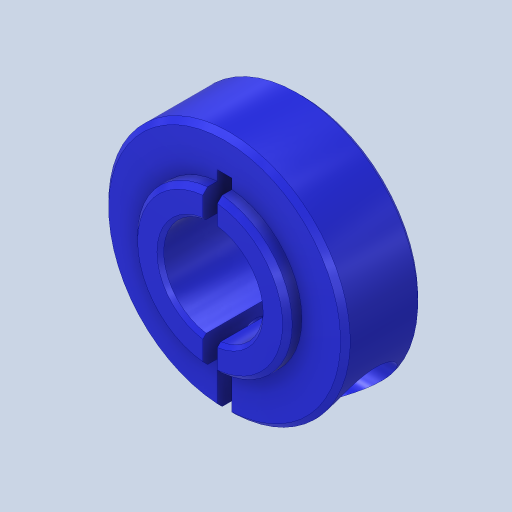
# Autodesk Inventor part: SCBNJ10-16b
Saved by Autodesk Inventor 2024 (Build 280153000, 153)
## iProperties
Category: PARTsolutions
Company: MISUMI
Created: 2024-03-13
Part Number: SCBNJ10-16b
Material: ABS プラスチック
Catalog Web Link: www.cadenas.de
Description: SCBNJ, PSCBNJ, SSCBNJ, SCSNAJ, SCSNAWJ, SCLSJ, PSCLSJ, SSCLSJ-b-Set Collars - For Bearing Fixing - Slit Compact Type
Vendor: MISUMI
Document SubType Name: Modeling
Designer: psAdmin
Manufacturer: MISUMI
Mass: 3.07278 g
Surface Area: 20.4444 cm^2
Volume: 3.07278 cm^3
Density: 1.06 g/cm^3
Appearance: 青 - 壁塗料 - 光沢
PSOL_IDENT_0: {$CADENAS_DATA/23d-libs/misumi/metric/03_set_collars/scbnj_b.prj},235 {VTYP=3D},{NB=SCBNJ10-16b},{LI
PSOL_IDENT_1: NA=SCBNJ10-16b},{NN=SCBNJ, PSCBNJ, SSCBNJ, SCSNAJ, SCSNAWJ, SCLSJ, PSCLSJ, SSCLSJ-b},{DATE=31.05.202
PSOL_IDENT_2: 3 07:34:13},{GEOMDATE=14.04.2023 07:53:48},{VERSION=},{LINEID=60},{WBVAR=TS,MAT,ST,DSS},{WBNUMERIC=D
PSOL_IDENT_3: SS}  {NB=SCBNJ10-16b},{LINA=SCBNJ10-16b},{KT=DUMMY},{PN=SCBNJ10-16},{TYPE=SCBNJ},{D=10},{TS=SN},{TS1='
PSOL_IDENT_4: SN','Short Nose','LN','Long Nose'},{MAT=1045},{MATA='1045','1045 Carbon Steel','304','304 Stainless
PSOL_IDENT_5: Steel','2017','2017 Aluminum Alloy'},{ST=Black Oxide},{ST0='Black Oxide','Black Oxide','Electroless
PSOL_IDENT_6: Nickel Plating','Electroless Nickel Plating'},{DSS=16},{DS1=13,14,16},{AC=Set Screws 2 Pcs.},{AB=620
PSOL_IDENT_7: 0ZZ(30)-6300ZZ(35)},{B=9.5},{B1=12.0},{D1=25},{M=M3},{THMD=3},{BB=8.0},{C=0.5},{L=10},{DD=3.5},{R=3.
PSOL_IDENT_8: 00},{W=1.5},{X=8.0},{Y=4.0},{Z=9.000},{COLOR=0.00,0.00,0.00,0.00}
NB: SCBNJ10-16b
NN: SCBNJ, PSCBNJ, SSCBNJ, SCSNAJ, SCSNAWJ, SCLSJ, PSCLSJ, SSCLSJ-b
NT: Set Collars - For Bearing Fixing - Slit Compact Type
NBSYN: $PN.b
LINA: SCBNJ10-16b
CATALOG: Misumi
PN: SCBNJ10-16
D: 10
TS: Short Nose
MAT: 1045 Carbon Steel
ST: Black Oxide
DSS: 16
AC: Set Screws 2 Pcs.
AB: 6200ZZ(30)-6300ZZ(35)
B: 9.5
B1: 12
D1: 25
M: M3
BB: 8
C: 0.5
L: 10
DD: 3.5
R: 3
W: 1.5
X: 8
Y: 4
Z: 9
SUPPLIER: MISUMI
ARTICLENO: SCBNJ10-16b
BOMINFO: SCBNJ10-16b
CREATOR: CADENAS GmbH
Title: SCBNJ10-16b
Author: Cadenas PARTsolutions
Comments: Set Collars - For Bearing Fixing - Slit Compact Type
Autodesk Inventor part; units mm, degrees
sketch "Sketch_1" plane through (0, 0, 0) normal (1, 0, 0) x (0, 1, 0)
  line L0 (0, -4) -> (0, 5.5)
  line L1 (7.5, 5.5) -> (5.5, 5.5)
  line L2 (5.5, 5.5) -> (5, 5)
  line L3 (5, 5) -> (5, -3.5)
  line L4 (5, -3.5) -> (5.5, -4)
  line L5 (5.5, -4) -> (12, -4)
  line L6 (12, -4) -> (12.5, -3.5)
  line L7 (12.5, -3.5) -> (12.5, 3.5)
  line L8 (12.5, 3.5) -> (12, 4)
  line L9 (12, 4) -> (8, 4)
  line L10 (8, 4) -> (8, 5)
  line L11 (8, 5) -> (7.5, 5.5)
  constraints: 24 end point
revolve "Revolution1" add sketch "Sketch_1" angle 360 about axis through (0, 0, -4) along (0, 0, -1)
sketch "Sketch_2" plane through (0, 0, 0) normal (0, 0, 1) x (1, 0, 0)
  line L0 (-0.75, -12.5) -> (0.75, -12.5)
  line L1 (0.75, -12.5) -> (0.75, 9)
  line L2 (0.75, 9) -> (-0.75, 9)
  line L3 (-0.75, 9) -> (-0.75, -12.5)
  constraints: 8 end point
extrude "Extrusion1" cut sketch "Sketch_2" along normal mid plane 32
sketch "Sketch_3" plane through (0, 0, 0) normal (0, 0, 1) x (1, 0, 0)
  line L0 (0, -8) -> (12.5, -8)
  line L1 (12.5, -8) -> (12.5, -11)
  line L2 (12.5, -11) -> (4, -11)
  line L3 (4, -11) -> (4, -9.75)
  line L4 (4, -9.75) -> (0, -9.75)
  line L5 (0, -9.75) -> (0, -8)
  line L6 (0, -8) -> (12.5, -8)
  constraints: 14 end point
ref_plane "body_screw_XY" through (4, -8, 0) normal (1, 0, 0) x (0, 0, -1)
ref_plane "body_screw_YZ" through (4, -8, 0) normal (0, 0, -1) x (0, 1, 0)
ref_plane "body_screw_ZX" through (4, -8, 0) normal (0, 1, 0) x (1, 0, 0)
ref_plane "作業平面5" through (4, -8, 0) normal (1, 0, 0) x (0, 0, -1)
sketch "スケッチ5" plane through (4, -8, 0) normal (1, 0, 0) x (0, 0, -1)
  point P0 (0, 8)
ref_plane "作業平面6" through (4, -8, 0) normal (1, 0, 0) x (0, 0, -1)
sketch "スケッチ6" plane through (4, -8, 0) normal (1, 0, 0) x (0, 0, -1)
  point P0 (0, 8)
sketch "スケッチ7" plane through (0, 0, -4) normal (0, 0, -1) x (-1, 0, 0)
  circle A0 centre (0, 0) radius 5.15
  dimension "d12" = 10.3
  constraints: 1 centre point, 1 coincident
  measures "d12" diameter of A0
extrude "押し出し2" cut sketch "スケッチ7" against normal blind 10
ref_plane "作業平面4" through (12.5, 0, 0) normal (1, 0, 0) x (0, 1, 0)
sketch "スケッチ8" plane through (12.5, 0, 0) normal (1, 0, 0) x (0, 1, 0)
  circle A0 centre (-8, 0) radius 1.75 projected
  circle A1 centre (-8, 0) radius 1.7
  circle A2 centre (-8, 0) radius 3.5
  point P0 (0, 0)
  dimension "d15" = 3.4
  dimension "d16" = 7
  constraints: 2 centre point, 2 coincident
  measures "d15" diameter of A1
  measures "d16" diameter of A2
extrude "押し出し3" cut sketch "スケッチ8" against normal through all contours A1
extrude "押し出し4" cut sketch "スケッチ8" against normal blind 8.5 contours A0 | A1 | A2
mirror "ミラー1" about plane through (0, 0, 0) normal (1, 0, 0) of "押し出し4"
body "Solid1"
